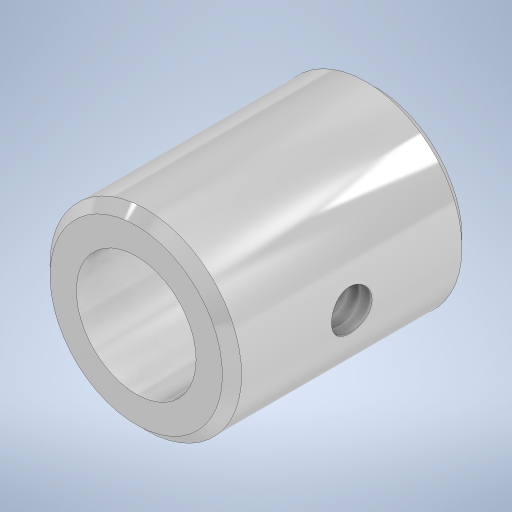
# Autodesk Inventor part: Carriage Axle Set Screw Holder
Saved by Autodesk Inventor 2023 (Build 270158000, 158)
## iProperties
Created: 2023-02-15
Part Number: Carriage Axle Set Screw Holder
Material: Generic
Document SubType Name: Modeling
Designer: mbear
Density: 1 g/cm^3
Appearance: Default
Author: mbear
Autodesk Inventor part; units mm, degrees
ref_plane "XZ Plane" through (0, 0, 0) normal (0, 1, 0) x (-1, 0, 0)
ref_plane "XY Plane" through (0, 0, 0) normal (0, 0, 1) x (1, 0, 0)
sketch "Sketch1" plane through (0, 0, 0) normal (0, 0, 1) x (1, 0, 0)
  circle A0 centre (0, 0) radius 3.175
  circle A1 centre (0, 0) radius 5.08
  dimension "d0" = 6.35
  dimension "d1" = 10.16
  constraints: 2 centre point, 2 coincident
  measures "d0" diameter of A0
  measures "d1" diameter of A1
extrude "Extrusion1" add sketch "Sketch1" along normal blind 12.7
chamfer "Chamfer1" distance 0.508 angle 45 2 edges at (-5.08, 0, 12.7) (-5.08, 0, 0)
ref_plane "Work Plane1" through (6.35, 0, 0) normal (1, 0, 0) x (0, 1, 0)
sketch "Sketch2" plane through (6.35, 0, 0) normal (1, 0, 0) x (0, 1, 0)
  circle A0 centre (0, 6.35) radius 1.1282
  point P0 (0, 0)
  dimension "d8" = 6.35
  constraints: 1 centre point, 1 vertical alignment
  measures "d8" distance of point (0, 0) A0.centre
hole "Hole1" at (6.35, 0, 6.35) direction (-1, 0, 0) diameter 2.1565 depth 6.35 thread size "4-40 UNC" class "2B" standard "ANSI Unified Screw Threads"
body "Solid1"
